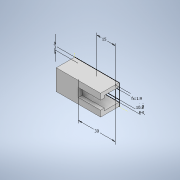
# Autodesk Inventor part: button_fix
Saved by Autodesk Inventor 2020 (Build 240168000, 168)
## iProperties
Created: 2022-09-29
Part Number: button_fix
Material: 일반
Document SubType Name: Modeling
Designer: taewo
Density: 1 g/cm^3
Appearance: 기본값
Author: taewo
Autodesk Inventor part; units mm, degrees
ref_plane "YZ Plane" through (0, 0, 0) normal (1, 0, 0) x (0, 1, 0)
ref_plane "XZ Plane" through (0, 0, 0) normal (0, 1, 0) x (-1, 0, 0)
ref_plane "XY Plane" through (0, 0, 0) normal (0, 0, 1) x (1, 0, 0)
sketch "sketch" plane through (0, 0, 0) normal (0, 0, 1) x (1, 0, 0)
  line L0 (-7.2, 0) -> (43.2, 0) construction
  line L1 (0, -3.36) -> (0, 20.16) construction
  line L2 (3, 13.8) -> (33, 13.8)
  line L3 (33, 13.8) -> (33, 3)
  line L4 (33, 3) -> (3, 3)
  line L5 (3, 3) -> (3, 13.8)
  line L6 (18, 11.9) -> (33, 11.9)
  line L7 (33, 11.9) -> (33, 4.9)
  line L8 (33, 4.9) -> (18, 4.9)
  line L9 (18, 4.9) -> (18, 11.9)
  line L10 (36, 16.8) -> (0, 16.8)
  line L11 (0, 16.8) -> (0, 0)
  line L12 (0, 0) -> (36, 0)
  line L13 (36, 0) -> (36, 16.8)
  line L14 (33, 4.9) -> (36, 4.9)
  line L15 (33, 11.9) -> (36, 11.9)
  line L16 (0, 3) -> (3, 3)
  line L17 (0, 13.8) -> (3, 13.8)
  line L18 (33, 3) -> (36, 3)
  line L19 (33, 13.8) -> (36, 13.8)
  dimension "d0" = 10.8
  dimension "d2" = 7
  dimension "d3" = 1.9
  dimension "d4" = 15
  dimension "d5" = 30
  dimension "d6" = 3
  constraints: 36 end point, 8 perpendicular, 7 parallel, 6 point on line, 2 horizontal, 1 collinear, 3 other
  measures "d0" distance of L2.end L3.end
  measures "d2" distance of L6.end L7.end
  measures "d3" distance between parallel lines of L2 L6
  measures "d4" distance of L6.start L6.end
  measures "d5" distance of L3.end L4.end
  measures "d6" distance between parallel lines of L2 L10
extrude "돌출1" add sketch "sketch" along normal blind 15
extrude "floor" cut sketch "sketch" along normal blind 12 contours L2 L3 L6 L9 L8 L4 L5 | L5 L16 L11 L17 | L19 L13 L15 L3 | L3 L14 L13 L18
extrude "fix" cut sketch "sketch" along normal up to surface (15 mm away) contours L15 L13 L14 L3 | L3 L8 L9 L6
equation "\"d3\" = -0.5 * d2 + 0.5 * d0"
